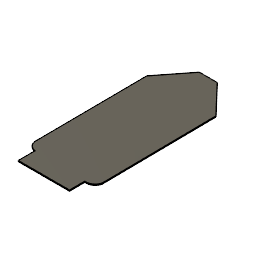
Case_outline (Autodesk Fusion 360 design; units mm, degrees)
part number: 2026-08-28-15-58-51-813
Autodesk Fusion 360 part; units mm, degrees
note: some values were not read from the file. Set by a fixed rule: which sketch regions a step uses.
sketch "KiCad Dongle-Edge_Cuts" plane through (0, 0, 0) normal (0, 1, 0) x (1, 0, 0)
  line L0 (143.0096, -51.9769) -> (143.0098, -51.9771)
  line L1 (143.0098, -51.9771) -> (143.0101, -51.9771)
  line L2 (143.0101, -51.9771) -> (143.0181, -51.9827)
  line L3 (143.0181, -51.9827) -> (154.0181, -63.4827)
  line L4 (154.0181, -63.4827) -> (154.0225, -63.4897)
  line L5 (154.0225, -63.4897) -> (154.023, -63.4902)
  line L6 (154.023, -63.4902) -> (154.0231, -63.4906)
  line L7 (154.0231, -63.4906) -> (154.0233, -63.4909)
  line L8 (154.0233, -63.4909) -> (154.0233, -63.4916)
  line L9 (154.0233, -63.4916) -> (154.025, -63.4997)
  line L10 (154.025, -63.4997) -> (154.525, -107.9997)
  line L11 (154.525, -107.9997) -> (154.5245, -108.0022)
  line L12 (154.5245, -108.0022) -> (154.5247, -108.0035)
  line L13 (154.5247, -108.0035) -> (154.4584, -108.3466)
  line L14 (154.4584, -108.3466) -> (154.3588, -108.6815)
  line L15 (154.3588, -108.6815) -> (154.2268, -109.005)
  line L16 (154.2268, -109.005) -> (154.0637, -109.3141)
  line L17 (154.0637, -109.3141) -> (153.8712, -109.6056)
  line L18 (153.8712, -109.6056) -> (153.651, -109.8769)
  line L19 (153.651, -109.8769) -> (153.4052, -110.1253)
  line L20 (153.4052, -110.1253) -> (153.1363, -110.3484)
  line L21 (153.1363, -110.3484) -> (152.8468, -110.5441)
  line L22 (152.8468, -110.5441) -> (152.5396, -110.7105)
  line L23 (152.5396, -110.7105) -> (152.2175, -110.8459)
  line L24 (152.2175, -110.8459) -> (151.8837, -110.9491)
  line L25 (151.8837, -110.9491) -> (151.5413, -111.0191)
  line L26 (151.5413, -111.0191) -> (151.1938, -111.0553)
  line L27 (151.1938, -111.0553) -> (150.8444, -111.0571)
  line L28 (150.8444, -111.0571) -> (150.525, -111.0274)
  line L29 (150.525, -111.0274) -> (150.525, -117)
  line L30 (150.525, -117) -> (150.5231, -117.0096)
  line L31 (150.5231, -117.0096) -> (150.5096, -117.0231)
  line L32 (150.5096, -117.0231) -> (150.5, -117.025)
  line L33 (150.5, -117.025) -> (134, -117.025)
  line L34 (134, -117.025) -> (130.5, -117.025)
  line L35 (130.5, -117.025) -> (130.4904, -117.0231)
  line L36 (130.4904, -117.0231) -> (130.4769, -117.0096)
  line L37 (130.4769, -117.0096) -> (130.475, -117)
  line L38 (130.475, -117) -> (130.475, -110.4205)
  line L39 (130.475, -110.4205) -> (130.1411, -110.3722)
  line L40 (130.1411, -110.3722) -> (129.7916, -110.2849)
  line L41 (129.7916, -110.2849) -> (129.4527, -110.1627)
  line L42 (129.4527, -110.1627) -> (129.1278, -110.0068)
  line L43 (129.1278, -110.0068) -> (128.8204, -109.819)
  line L44 (128.8204, -109.819) -> (128.5336, -109.601)
  line L45 (128.5336, -109.601) -> (128.2702, -109.3552)
  line L46 (128.2702, -109.3552) -> (128.033, -109.084)
  line L47 (128.033, -109.084) -> (127.8245, -108.7902)
  line L48 (127.8245, -108.7902) -> (127.6467, -108.4768)
  line L49 (127.6467, -108.4768) -> (127.5015, -108.1471)
  line L50 (127.5015, -108.1471) -> (127.3903, -107.8044)
  line L51 (127.3903, -107.8044) -> (127.3144, -107.4522)
  line L52 (127.3144, -107.4522) -> (127.2744, -107.0942)
  line L53 (127.2744, -107.0942) -> (127.2708, -106.7339)
  line L54 (127.2708, -106.7339) -> (127.3034, -106.378)
  line L55 (127.3034, -106.378) -> (126.975, -63.5002)
  line L56 (126.975, -63.5002) -> (126.9761, -63.4946)
  line L57 (126.9761, -63.4946) -> (126.9759, -63.4933)
  line L58 (126.9759, -63.4933) -> (126.9766, -63.492)
  line L59 (126.9766, -63.492) -> (126.9768, -63.4906)
  line L60 (126.9768, -63.4906) -> (126.9777, -63.4897)
  line L61 (126.9777, -63.4897) -> (126.9803, -63.4846)
  line L62 (126.9803, -63.4846) -> (135.9803, -51.9846)
  line L63 (135.9803, -51.9846) -> (135.9877, -51.9782)
  line L64 (135.9877, -51.9782) -> (135.9893, -51.978)
  line L65 (135.9893, -51.978) -> (135.9904, -51.9769)
  line L66 (135.9904, -51.9769) -> (136, -51.975)
  line L67 (136, -51.975) -> (143, -51.975)
  line L68 (143, -51.975) -> (143.0096, -51.9769)
  line L69 (136.0122, -52.025) -> (127.0251, -63.5085)
  line L70 (127.0251, -63.5085) -> (127.3534, -106.3785)
  line L71 (127.3534, -106.3785) -> (127.353, -106.3809)
  line L72 (127.353, -106.3809) -> (127.3532, -106.3822)
  line L73 (127.3532, -106.3822) -> (127.328, -106.5583)
  line L74 (127.328, -106.5583) -> (127.3136, -106.9136)
  line L75 (127.3136, -106.9136) -> (127.3351, -107.2687)
  line L76 (127.3351, -107.2687) -> (127.3924, -107.6197)
  line L77 (127.3924, -107.6197) -> (127.4849, -107.9631)
  line L78 (127.4849, -107.9631) -> (127.6116, -108.2955)
  line L79 (127.6116, -108.2955) -> (127.7712, -108.6133)
  line L80 (127.7712, -108.6133) -> (127.9621, -108.9134)
  line L81 (127.9621, -108.9134) -> (128.1824, -109.1926)
  line L82 (128.1824, -109.1926) -> (128.4298, -109.4482)
  line L83 (128.4298, -109.4482) -> (128.7018, -109.6774)
  line L84 (128.7018, -109.6774) -> (128.9955, -109.878)
  line L85 (128.9955, -109.878) -> (129.308, -110.0479)
  line L86 (129.308, -110.0479) -> (129.636, -110.1853)
  line L87 (129.636, -110.1853) -> (129.9763, -110.2889)
  line L88 (129.9763, -110.2889) -> (130.3253, -110.3575)
  line L89 (130.3253, -110.3575) -> (130.5023, -110.374)
  line L90 (130.5023, -110.374) -> (130.5065, -110.3758)
  line L91 (130.5065, -110.3758) -> (130.5096, -110.3758)
  line L92 (130.5096, -110.3758) -> (130.5119, -110.3782)
  line L93 (130.5119, -110.3782) -> (130.5165, -110.3802)
  line L94 (130.5165, -110.3802) -> (130.5203, -110.3866)
  line L95 (130.5203, -110.3866) -> (130.5231, -110.3894)
  line L96 (130.5231, -110.3894) -> (130.5237, -110.3922)
  line L97 (130.5237, -110.3922) -> (130.5244, -110.3934)
  line L98 (130.5244, -110.3934) -> (130.5242, -110.3951)
  line L99 (130.5242, -110.3951) -> (130.525, -110.3989)
  line L100 (130.525, -110.3989) -> (130.525, -116.975)
  line L101 (130.525, -116.975) -> (134, -116.975)
  line L102 (134, -116.975) -> (150.475, -116.975)
  line L103 (150.475, -116.975) -> (150.475, -111)
  line L104 (150.475, -111) -> (150.4769, -110.9904)
  line L105 (150.4769, -110.9904) -> (150.4774, -110.9899)
  line L106 (150.4774, -110.9899) -> (150.4776, -110.989)
  line L107 (150.4776, -110.989) -> (150.4883, -110.9779)
  line L108 (150.4883, -110.9779) -> (150.4897, -110.9777)
  line L109 (150.4897, -110.9777) -> (150.4904, -110.9769)
  line L110 (150.4904, -110.9769) -> (150.494, -110.9769)
  line L111 (150.494, -110.9769) -> (150.5035, -110.9753)
  line L112 (150.5035, -110.9753) -> (150.6743, -110.9996)
  line L113 (150.6743, -110.9996) -> (151.0189, -111.0147)
  line L114 (151.0189, -111.0147) -> (151.3633, -110.9959)
  line L115 (151.3633, -110.9959) -> (151.7042, -110.9435)
  line L116 (151.7042, -110.9435) -> (152.0383, -110.8579)
  line L117 (152.0383, -110.8579) -> (152.3624, -110.74)
  line L118 (152.3624, -110.74) -> (152.6735, -110.5908)
  line L119 (152.6735, -110.5908) -> (152.9684, -110.4119)
  line L120 (152.9684, -110.4119) -> (153.2443, -110.205)
  line L121 (153.2443, -110.2049) -> (153.4986, -109.9719)
  line L122 (153.4986, -109.9719) -> (153.7289, -109.7151)
  line L123 (153.7289, -109.7151) -> (153.9329, -109.437)
  line L124 (153.9329, -109.437) -> (154.1086, -109.1402)
  line L125 (154.1086, -109.1402) -> (154.2544, -108.8276)
  line L126 (154.2544, -108.8276) -> (154.3688, -108.5022)
  line L127 (154.3688, -108.5022) -> (154.4509, -108.1672)
  line L128 (154.4509, -108.1672) -> (154.475, -107.9984)
  line L129 (154.475, -107.9984) -> (153.9751, -63.5101)
  line L130 (153.9751, -63.5101) -> (142.9893, -52.025)
  line L131 (142.9893, -52.025) -> (136.0122, -52.025)
sketch "KiCad Dongle-Edge_Cuts (1)" plane through (0, 0, 0) normal (0, 0, 1) x (1, 0, 0)
  line L0 (143.0096, -51.9769) -> (143.0098, -51.9771)
  line L1 (143.0098, -51.9771) -> (143.0101, -51.9771)
  line L2 (143.0101, -51.9771) -> (143.0181, -51.9827)
  line L3 (143.0181, -51.9827) -> (154.0181, -63.4827)
  line L4 (154.0181, -63.4827) -> (154.0225, -63.4897)
  line L5 (154.0225, -63.4897) -> (154.023, -63.4902)
  line L6 (154.023, -63.4902) -> (154.0231, -63.4906)
  line L7 (154.0231, -63.4906) -> (154.0233, -63.4909)
  line L8 (154.0233, -63.4909) -> (154.0233, -63.4916)
  line L9 (154.0233, -63.4916) -> (154.025, -63.4997)
  line L10 (154.025, -63.4997) -> (154.525, -107.9997)
  line L11 (154.525, -107.9997) -> (154.5245, -108.0022)
  line L12 (154.5245, -108.0022) -> (154.5247, -108.0035)
  line L13 (154.5247, -108.0035) -> (154.4584, -108.3466)
  line L14 (154.4584, -108.3466) -> (154.3588, -108.6815)
  line L15 (154.3588, -108.6815) -> (154.2268, -109.005)
  line L16 (154.2268, -109.005) -> (154.0637, -109.3141)
  line L17 (154.0637, -109.3141) -> (153.8712, -109.6056)
  line L18 (153.8712, -109.6056) -> (153.651, -109.8769)
  line L19 (153.651, -109.8769) -> (153.4052, -110.1253)
  line L20 (153.4052, -110.1253) -> (153.1363, -110.3484)
  line L21 (153.1363, -110.3484) -> (152.8468, -110.5441)
  line L22 (152.8468, -110.5441) -> (152.5396, -110.7105)
  line L23 (152.5396, -110.7105) -> (152.2175, -110.8459)
  line L24 (152.2175, -110.8459) -> (151.8837, -110.9491)
  line L25 (151.8837, -110.9491) -> (151.5413, -111.0191)
  line L26 (151.5413, -111.0191) -> (151.1938, -111.0553)
  line L27 (151.1938, -111.0553) -> (150.8444, -111.0571)
  line L28 (150.8444, -111.0571) -> (150.525, -111.0274)
  line L29 (150.525, -111.0274) -> (150.525, -117)
  line L30 (150.525, -117) -> (150.5231, -117.0096)
  line L31 (150.5231, -117.0096) -> (150.5096, -117.0231)
  line L32 (150.5096, -117.0231) -> (150.5, -117.025)
  line L33 (150.5, -117.025) -> (134, -117.025)
  line L34 (134, -117.025) -> (130.5, -117.025)
  line L35 (130.5, -117.025) -> (130.4904, -117.0231)
  line L36 (130.4904, -117.0231) -> (130.4769, -117.0096)
  line L37 (130.4769, -117.0096) -> (130.475, -117)
  line L38 (130.475, -117) -> (130.475, -110.4205)
  line L39 (130.475, -110.4205) -> (130.1411, -110.3722)
  line L40 (130.1411, -110.3722) -> (129.7916, -110.2849)
  line L41 (129.7916, -110.2849) -> (129.4527, -110.1627)
  line L42 (129.4527, -110.1627) -> (129.1278, -110.0068)
  line L43 (129.1278, -110.0068) -> (128.8204, -109.819)
  line L44 (128.8204, -109.819) -> (128.5336, -109.601)
  line L45 (128.5336, -109.601) -> (128.2702, -109.3552)
  line L46 (128.2702, -109.3552) -> (128.033, -109.084)
  line L47 (128.033, -109.084) -> (127.8245, -108.7902)
  line L48 (127.8245, -108.7902) -> (127.6467, -108.4768)
  line L49 (127.6467, -108.4768) -> (127.5015, -108.1471)
  line L50 (127.5015, -108.1471) -> (127.3903, -107.8044)
  line L51 (127.3903, -107.8044) -> (127.3144, -107.4522)
  line L52 (127.3144, -107.4522) -> (127.2744, -107.0942)
  line L53 (127.2744, -107.0942) -> (127.2708, -106.7339)
  line L54 (127.2708, -106.7339) -> (127.3034, -106.378)
  line L55 (127.3034, -106.378) -> (126.975, -63.5002)
  line L56 (126.975, -63.5002) -> (126.9761, -63.4946)
  line L57 (126.9761, -63.4946) -> (126.9759, -63.4933)
  line L58 (126.9759, -63.4933) -> (126.9766, -63.492)
  line L59 (126.9766, -63.492) -> (126.9768, -63.4906)
  line L60 (126.9768, -63.4906) -> (126.9777, -63.4897)
  line L61 (126.9777, -63.4897) -> (126.9803, -63.4846)
  line L62 (126.9803, -63.4846) -> (135.9803, -51.9846)
  line L63 (135.9803, -51.9846) -> (135.9877, -51.9782)
  line L64 (135.9877, -51.9782) -> (135.9893, -51.978)
  line L65 (135.9893, -51.978) -> (135.9904, -51.9769)
  line L66 (135.9904, -51.9769) -> (136, -51.975)
  line L67 (136, -51.975) -> (143, -51.975)
  line L68 (143, -51.975) -> (143.0096, -51.9769)
  line L69 (136.0122, -52.025) -> (127.0251, -63.5085)
  line L70 (127.0251, -63.5085) -> (127.3534, -106.3785)
  line L71 (127.3534, -106.3785) -> (127.353, -106.3809)
  line L72 (127.353, -106.3809) -> (127.3532, -106.3822)
  line L73 (127.3532, -106.3822) -> (127.328, -106.5583)
  line L74 (127.328, -106.5583) -> (127.3136, -106.9136)
  line L75 (127.3136, -106.9136) -> (127.3351, -107.2687)
  line L76 (127.3351, -107.2687) -> (127.3924, -107.6197)
  line L77 (127.3924, -107.6197) -> (127.4849, -107.9631)
  line L78 (127.4849, -107.9631) -> (127.6116, -108.2955)
  line L79 (127.6116, -108.2955) -> (127.7712, -108.6133)
  line L80 (127.7712, -108.6133) -> (127.9621, -108.9134)
  line L81 (127.9621, -108.9134) -> (128.1824, -109.1926)
  line L82 (128.1824, -109.1926) -> (128.4298, -109.4482)
  line L83 (128.4298, -109.4482) -> (128.7018, -109.6774)
  line L84 (128.7018, -109.6774) -> (128.9955, -109.878)
  line L85 (128.9955, -109.878) -> (129.308, -110.0479)
  line L86 (129.308, -110.0479) -> (129.636, -110.1853)
  line L87 (129.636, -110.1853) -> (129.9763, -110.2889)
  line L88 (129.9763, -110.2889) -> (130.3253, -110.3575)
  line L89 (130.3253, -110.3575) -> (130.5023, -110.374)
  line L90 (130.5023, -110.374) -> (130.5065, -110.3758)
  line L91 (130.5065, -110.3758) -> (130.5096, -110.3758)
  line L92 (130.5096, -110.3758) -> (130.5119, -110.3782)
  line L93 (130.5119, -110.3782) -> (130.5165, -110.3802)
  line L94 (130.5165, -110.3802) -> (130.5203, -110.3866)
  line L95 (130.5203, -110.3866) -> (130.5231, -110.3894)
  line L96 (130.5231, -110.3894) -> (130.5237, -110.3922)
  line L97 (130.5237, -110.3922) -> (130.5244, -110.3934)
  line L98 (130.5244, -110.3934) -> (130.5242, -110.3951)
  line L99 (130.5242, -110.3951) -> (130.525, -110.3989)
  line L100 (130.525, -110.3989) -> (130.525, -116.975)
  line L101 (130.525, -116.975) -> (134, -116.975)
  line L102 (134, -116.975) -> (150.475, -116.975)
  line L103 (150.475, -116.975) -> (150.475, -111)
  line L104 (150.475, -111) -> (150.4769, -110.9904)
  line L105 (150.4769, -110.9904) -> (150.4774, -110.9899)
  line L106 (150.4774, -110.9899) -> (150.4776, -110.989)
  line L107 (150.4776, -110.989) -> (150.4883, -110.9779)
  line L108 (150.4883, -110.9779) -> (150.4897, -110.9777)
  line L109 (150.4897, -110.9777) -> (150.4904, -110.9769)
  line L110 (150.4904, -110.9769) -> (150.494, -110.9769)
  line L111 (150.494, -110.9769) -> (150.5035, -110.9753)
  line L112 (150.5035, -110.9753) -> (150.6743, -110.9996)
  line L113 (150.6743, -110.9996) -> (151.0189, -111.0147)
  line L114 (151.0189, -111.0147) -> (151.3633, -110.9959)
  line L115 (151.3633, -110.9959) -> (151.7042, -110.9435)
  line L116 (151.7042, -110.9435) -> (152.0383, -110.8579)
  line L117 (152.0383, -110.8579) -> (152.3624, -110.74)
  line L118 (152.3624, -110.74) -> (152.6735, -110.5908)
  line L119 (152.6735, -110.5908) -> (152.9684, -110.4119)
  line L120 (152.9684, -110.4119) -> (153.2443, -110.205)
  line L121 (153.2443, -110.2049) -> (153.4986, -109.9719)
  line L122 (153.4986, -109.9719) -> (153.7289, -109.7151)
  line L123 (153.7289, -109.7151) -> (153.9329, -109.437)
  line L124 (153.9329, -109.437) -> (154.1086, -109.1402)
  line L125 (154.1086, -109.1402) -> (154.2544, -108.8276)
  line L126 (154.2544, -108.8276) -> (154.3688, -108.5022)
  line L127 (154.3688, -108.5022) -> (154.4509, -108.1672)
  line L128 (154.4509, -108.1672) -> (154.475, -107.9984)
  line L129 (154.475, -107.9984) -> (153.9751, -63.5101)
  line L130 (153.9751, -63.5101) -> (142.9893, -52.025)
  line L131 (142.9893, -52.025) -> (136.0122, -52.025)
extrude "Extrude2" add sketch "KiCad Dongle-Edge_Cuts (1)" along normal blind 0.4 contours L69 L70 L71 L73 L74 L75 L76 L77 L78 L79 L80 L81 L82 L83 L84 L85 L86 L87 L88 L89 L90 L91 L92 L93 L94 L95 L96 L98 L99 L100 L101 L102 L103 L104 L107 L109 L110 L111 L112 L113 L114 L115 L116 L117 L118 L119 L120 L121 L122 L123 L124 L125 L126 L127 L128 L129 L130 L131
